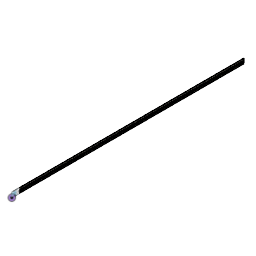
model_almost_done (Autodesk Fusion 360 archive; units mm, degrees)
design "Striscia_led"
Autodesk Fusion 360 part; units mm, degrees
sketch "Schizzo1" plane through (0, 0, 0) normal (1, 0, 0) x (0, 1, 0)
  line L0 (0, 0) -> (12.6, 0)
  line L1 (12.6, 0) -> (12.6, 9.55)
  line L2 (12.6, 9.55) -> (0, 9.55)
  line L3 (0, 9.55) -> (0, 0)
  line L4 (9.25, 6.55) -> (11.9, 6.55)
  line L5 (11.9, 6.55) -> (11.9, 3)
  line L6 (11.9, 3) -> (9.25, 3)
  line L7 (9.25, 3) -> (9.25, 6.55)
  line L8 (4.8, 6.55) -> (7.45, 6.55)
  line L9 (7.45, 6.55) -> (7.45, 3)
  line L10 (7.45, 3) -> (4.8, 3)
  line L11 (4.8, 3) -> (4.8, 6.55)
  line L12 (0.8, 6.55) -> (3.45, 6.55)
  line L13 (3.45, 6.55) -> (3.45, 3)
  line L14 (3.45, 3) -> (0.8, 3)
  line L15 (0.8, 3) -> (0.8, 6.55)
  dimension "d1" = 12.6
  dimension "d2" = 9.55
  dimension "d3" = 3.55
  dimension "d4" = 2.65
  dimension "d5" = 3
  dimension "d6" = 0.7
  dimension "d7" = 3.55
  dimension "d8" = 2.65
  dimension "d11" = 3.55
  dimension "d12" = 2.65
  dimension "d14" = 1.8
  dimension "d15" = 1.35
  constraint horizontal L0
  constraint vertical L1
  constraint horizontal L2
  constraint vertical L3
  constraint coincident L0.start L3.end
  constraint horizontal L4
  constraint vertical L5
  constraint horizontal L6
  constraint vertical L7
  constraint horizontal L8
  constraint vertical L9
  constraint horizontal L10
  constraint vertical L11
  constraint horizontal L12
  constraint vertical L13
  constraint horizontal L14
  constraint vertical L15
  measures "d1" distance of L0.start L0.end
  measures "d2" distance of L0.start L2.end
  measures "d3" distance of L4.start L6.end
  measures "d4" distance of L5.end L6.end
  measures "d5" distance of L0 L6
  measures "d6" distance of L1 L5
  measures "d7" distance of L8.start L10.end
  measures "d8" distance of L9.end L10.end
  measures "d11" distance of L12.start L14.end
  measures "d12" distance of L13.end L14.end
  measures "d14" distance of L7 L9
  measures "d15" distance of L11 L13
extrude "Estrusione1" add sketch "Schizzo1" against normal blind 0.4 contours L0 L1 L2 L3 | L4 L5 L6 L7 | L8 L9 L10 L11 | L12 L13 L14 L15 makes body 1
extrude "Estrusione2" add sketch "Schizzo1" along normal blind 0.7 contours L4 L5 L6 L7 | L8 L9 L10 L11 | L12 L13 L14 L15 bodies 1
pattern_linear "Serie R1" count 37 spacing 12.6 along (0, 1, 0) of bodies 1 makes body 2 at (-0.4, 16.8, 6.3667) makes body 3 at (-0.4, 29.4, 6.3667) makes body 4 at (-0.4, 42, 3.1833) makes body 5 at (-0.4, 54.6, 6.3667) makes body 6 at (-0.4, 67.2, 6.3667) makes body 7 at (-0.4, 79.8, 6.3667) makes body 8 at (-0.4, 92.4, 6.3667) makes body 9 at (-0.4, 105, 6.3667) makes body 10 at (-0.4, 117.6, 6.3667) makes body 11 at (-0.4, 130.2, 6.3667) makes body 12 at (-0.4, 142.8, 6.3667) makes body 13 at (-0.4, 155.4, 6.3667) makes body 14 at (-0.4, 168, 6.3667) makes body 15 at (-0.4, 180.6, 6.3667) makes body 16 at (-0.4, 193.2, 6.3667) makes body 17 at (-0.4, 205.8, 6.3667) makes body 18 at (-0.4, 218.4, 6.3667) makes body 19 at (-0.4, 231, 6.3667) makes body 20 at (-0.4, 243.6, 6.3667) makes body 21 at (-0.4, 256.2, 3.1833) makes body 22 at (-0.4, 268.8, 3.1833) makes body 23 at (-0.4, 281.4, 3.1833) makes body 24 at (-0.4, 294, 3.1833) makes body 25 at (-0.4, 306.6, 3.1833) makes body 26 at (-0.4, 319.2, 3.1833) makes body 27 at (-0.4, 331.8, 3.1833) makes body 28 at (-0.4, 344.4, 3.1833) makes body 29 at (-0.4, 357, 3.1833) makes body 30 at (-0.4, 369.6, 3.1833) makes body 31 at (-0.4, 382.2, 3.1833) makes body 32 at (-0.4, 394.8, 3.1833) makes body 33 at (-0.4, 407.4, 3.1833) makes body 34 at (-0.4, 420, 3.1833) makes body 35 at (-0.4, 432.6, 3.1833) makes body 36 at (-0.4, 445.2, 3.1833) makes body 37 at (-0.4, 457.8, 3.1833)
combine "Combina1" operation add target body 1 tool bodies 8 20 3 4 13 36 18 22 11 25 15 30 2 26 10 34 19 32 27 14 24 12 31 9 29 17 7 21 33 5 16 6 23 28 37 35
equation "d3 = 3.25 mm + 0.3 mm"
equation "d7 = 3.25 mm + 0.3 mm"
equation "d11 = 3.25 mm + 0.3 mm"
equation "d18 = 1.1 mm - 0.4 mm"
